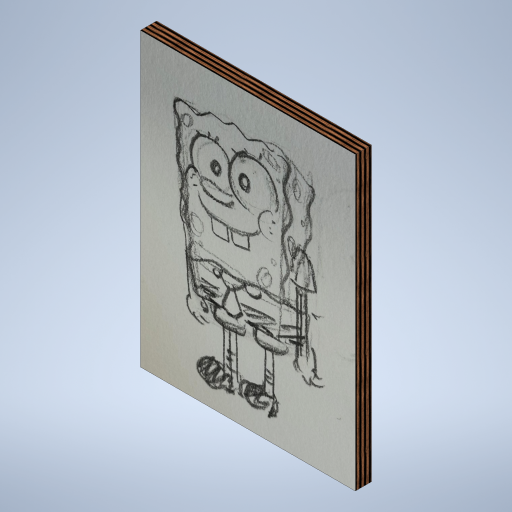
# Autodesk Inventor part: spong
Saved by Autodesk Inventor 2023 (Build 270158000, 158)
## iProperties
Created: 2024-07-02
Part Number: spong
Material: Generic
Document SubType Name: Modeling
Designer: Student-27
Density: 1 g/cm^3
Appearance: Default
Author: Student-27
Autodesk Inventor part; units mm, degrees
ref_plane "YZ Plane" through (0, 0, 0) normal (1, 0, 0) x (0, 1, 0)
ref_plane "XZ Plane" through (0, 0, 0) normal (0, 1, 0) x (-1, 0, 0)
ref_plane "XY Plane" through (0, 0, 0) normal (0, 0, 1) x (1, 0, 0)
sketch "Sketch1" plane through (0, 0, 0) normal (0, 0, 1) x (1, 0, 0)
  line L0 (-12.238, 10.3036) -> (787.862, 10.3036) construction
  line L1 (787.862, 10.3036) -> (787.862, -1056.4965) construction
  line L2 (787.862, -1056.4965) -> (-12.238, -1056.4965) construction
  line L3 (-12.238, -1056.4965) -> (-12.238, 10.3036) construction
  line L4 (227.1152, -318.4984) -> (563.3799, -318.4984)
  line L5 (563.3799, -318.4984) -> (563.3799, -774.7171)
  line L6 (563.3799, -774.7171) -> (227.1152, -774.7171)
  line L7 (227.1152, -774.7171) -> (227.1152, -318.4984)
  point P0 (0, 0)
  dimension "d3" = 336.2647
  dimension "d6" = 456.2187
  constraints: 8 end point, 2 parallel, 1 horizontal, 1 perpendicular, 2 other
  measures "d3" distance of L4.start L4.end
  measures "d6" distance of L6.end L4.start
extrude "Extrusion1" add sketch "Sketch1" against normal blind 25.4
body "Solid1"
